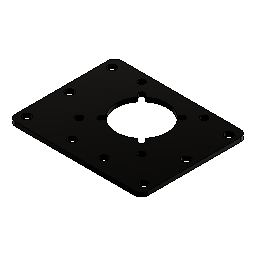
Router Concept v20 (Autodesk Fusion 360 archive; units mm, degrees)
design "Drive Module Bracket"
Autodesk Fusion 360 part; units mm, degrees
sketch "Dimension" plane through (0, 0, 0) normal (0, 1, 0) x (1, 0, 0)
  line L0 (50, -40) -> (-50, -40)
  line L1 (-50, -40) -> (-50, 40)
  line L2 (-50, 40) -> (50, 40)
  line L3 (50, 40) -> (50, -40)
  line L4 (50, -40) -> (-50, 40) construction
  line L5 (-50, -40) -> (50, 40) construction
  dimension "d4" = 100
  dimension "d5" = 80
  constraint horizontal L0
  constraint perpendicular L0 L1
  constraint parallel L0 L2
  constraint parallel L1 L3
  constraint coincident L4 origin
  constraint coincident L5 origin
  measures "d4" distance of L1.end L2.end
  measures "d5" distance of L0.end L1.end
extrude "Extrude1" add sketch "Dimension" along normal blind 3
sketch "Stepper Mount" plane through (0, 3, 0) normal (0, 1, 0) x (-1, 0, 0)
  line L0 (-50, -40) -> (50, -40)
  line L1 (50, -40) -> (50, 40)
  line L2 (50, 40) -> (-50, 40)
  line L3 (-50, 40) -> (-50, -40)
  line L4 (30, -40) -> (-30, -40)
  line L5 (-30, -40) -> (-30, 40) construction
  line L6 (-30, 40) -> (30, 40)
  line L7 (30, 40) -> (30, -40) construction
  circle A0 centre (23.55, -33.85) radius 2.55
  circle A1 centre (-23.55, -33.85) radius 2.55
  circle A2 centre (23.55, 13.25) radius 2.55
  circle A3 centre (-23.55, 13.25) radius 2.55
  line L8 (-23.55, 13.25) -> (23.55, -33.85)
  circle A4 centre (15.49, -25.79) radius 2
  line L9 (0, -10.3) -> (-30, -10.3) construction
  line L10 (0, -10.3) -> (0, -40) construction
  circle A5 centre (-15.49, -25.79) radius 2
  line L11 (15.49, -25.79) -> (-15.49, 5.19)
  line L12 (-15.49, 5.19) -> (-16.9042, 3.7758) construction
  line L13 (-16.9042, 3.7758) -> (14.0758, -27.2042)
  line L14 (14.0758, -27.2042) -> (15.49, -25.79)
  line L15 (15.49, -25.79) -> (-15.49, 5.19)
  line L16 (-15.49, 5.19) -> (-14.0758, 6.6042) construction
  line L17 (-14.0758, 6.6042) -> (16.9042, -24.3758)
  line L18 (16.9042, -24.3758) -> (15.49, -25.79)
  line L19 (14.0758, 6.6042) -> (-16.9042, -24.3758)
  line L20 (16.9042, 3.7758) -> (-14.0758, -27.2042)
  line L21 (23.55, 13.25) -> (13.5057, 3.2057) construction
  line L22 (1.4142, -8.8858) -> (-23.55, -33.85) construction
  arc A6 (16.9042, 3.7758) -> (14.0758, 6.6042) centre (15.49, 5.19) ccw
  arc A7 (-14.0758, 6.6042) -> (-16.9042, 3.7758) centre (-15.49, 5.19) ccw
  arc A8 (-13.5057, 3.2057) -> (-12.0173, 4.5457) centre (0, -10.3) ccw
  dimension "d8" = 60
  dimension "d9" = 38.2
  dimension "d10" = 30
  dimension "d11" = 29.7
  dimension "d12" = 5.1
  dimension "d13" = 6.45
  dimension "d14" = 6.15
  dimension "d15" = 5.1
  dimension "d16" = 6.15
  dimension "d17" = 53.55
  dimension "d18" = 5.1
  dimension "d19" = 6.45
  dimension "d20" = 53.25
  dimension "d21" = 5.1
  dimension "d22" = 53.25
  dimension "d23" = 53.55
  dimension "d24" = 14.51
  dimension "d25" = 14.21
  dimension "d26" = 4
  dimension "d27" = 2
  dimension "d28" = 2
  constraint horizontal L4
  constraint vertical L5
  constraint horizontal L6
  constraint vertical L7
  constraint midpoint L0 L4
  constraint collinear L2 L6
  constraint coincident A2.centre L21.start
  constraint coincident A1.centre L22.end
  constraint coincident A3.centre L8.start
  constraint coincident A0.centre L8.end
  constraint coincident L9.start L10.start
  constraint coincident L5 L9.end
  constraint perpendicular L5 L9
  constraint midpoint L4 L10.end
  constraint symmetric A4 L10 A5
  constraint symmetric A4 L9 A6
  constraint symmetric L9 A5 A7
  constraint perpendicular L11 L12
  constraint parallel L11 L13
  constraint parallel L12 L14
  constraint coincident L11.end L12.start
  constraint parallel L8 L11
  constraint coincident A4.centre L11.start
  constraint perpendicular L15 L16
  constraint parallel L15 L17
  constraint parallel L16 L18
  constraint perpendicular L12 L15
  constraint symmetric L10 L12.end L20.start
  constraint symmetric L10 L13.end L20.end
  constraint symmetric L10 L16.end L19.start
  constraint symmetric L10 L17.end L19.end
  constraint coincident L21.end A8
  constraint coincident L17 L22.start
  constraint collinear L21 L22
  constraint coincident L17 A8.end
  constraint coincident L8 A8.start
  measures "d8" distance of L4.start L4.end
  measures "d9" diameter of A8
  measures "d10" distance of L7 L9.start
  measures "d11" distance of L4 L9.start
  measures "d12" diameter of A0
  measures "d13" distance of L7 A0.centre
  measures "d14" distance of L4 A0.centre
  measures "d15" diameter of A1
  measures "d16" distance of L4 A1.centre
  measures "d17" distance of L7 A1.centre
  measures "d18" diameter of A2
  measures "d19" distance of L7 A2.centre
  measures "d20" distance of L4 A2.centre
  measures "d21" diameter of A3
  measures "d22" distance of L4 A3.centre
  measures "d23" distance of L7 A3.centre
  measures "d24" distance of L7 A4.centre
  measures "d25" distance of L4 A4.centre
  measures "d26" diameter of A4
  measures "d27" distance of A4.centre L13.end
  measures "d28" distance of A4.centre L17.end
extrude "Extrude2" cut sketch "Stepper Mount" against normal through all contours A0 | A1 | A2 | A3 | L8 L11 L15 L17 L19 A7 | L8 L11 L13 L15 A7 A8 | L8 L11 L13 L15 L19 A8 | L8 L11 L15 L17 L19 L20 | L8 L11 L13 L15 L19 L20 | L13 L19 A8 | L8 L11 L15 L17 L20 A8 | L8 L11 L13 L15 L20 A8 | L17 L19 L20 A8 | L17 L19 A8 | L13 L19 L20 A8 | A5 L19 L20 A8 | L8 A4 L11 L15 L17 A8 | L8 A4 L11 L13 L15 A8 | L17 L20 A8 | L13 L20 A8 | L19 L20 A6 A8 | A5 | L8 A4 L11 L15 L18 | L8 A4 L11 L14 L15 | L8 A4 L18 | L8 A4 L14
sketch "Idler Mount" plane through (0, 3, 0) normal (0, 1, 0) x (-1, 0, 0)
  circle A0 centre (23.55, 13.25) radius 2.55
  circle A1 centre (23.55, -33.85) radius 2.55
  line L0 (14.8457, -22.3173) -> (16.9042, -24.3758)
  arc A2 (14.0758, -27.2042) -> (16.9042, -24.3758) centre (15.49, -25.79) ccw
  line L1 (14.0758, -27.2042) -> (12.0173, -25.1457)
  arc A3 (-12.0173, -25.1457) -> (12.0173, -25.1457) centre (0, -10.3) ccw
  line L2 (-12.0173, -25.1457) -> (-14.0758, -27.2042)
  arc A4 (-16.9042, -24.3758) -> (-14.0758, -27.2042) centre (-15.49, -25.79) ccw
  line L3 (-16.9042, -24.3758) -> (-14.8457, -22.3173)
  arc A5 (-14.8457, 1.7173) -> (-14.8457, -22.3173) centre (0, -10.3) ccw
  line L4 (-14.8457, 1.7173) -> (-16.9042, 3.7758)
  arc A6 (-14.0758, 6.6042) -> (-16.9042, 3.7758) centre (-15.49, 5.19) ccw
  line L5 (-14.0758, 6.6042) -> (-12.0173, 4.5457)
  arc A7 (12.0173, 4.5457) -> (-12.0173, 4.5457) centre (0, -10.3) ccw
  line L6 (12.0173, 4.5457) -> (14.0758, 6.6042)
  arc A8 (16.9042, 3.7758) -> (14.0758, 6.6042) centre (15.49, 5.19) ccw
  line L7 (16.9042, 3.7758) -> (14.8457, 1.7173)
  arc A9 (14.8457, -22.3173) -> (14.8457, 1.7173) centre (0, -10.3) ccw
  circle A10 centre (-23.55, 13.25) radius 2.55
  circle A11 centre (-23.55, -33.85) radius 2.55
  line L8 (-50, -40) -> (50, -40)
  line L9 (50, -40) -> (50, 40)
  line L10 (50, 40) -> (-50, 40)
  line L11 (-50, 40) -> (-50, -40)
  arc A12 (-14.8457, 1.7173) -> (-14.8457, -22.3173) centre (0, -10.3) ccw
  arc A13 (-12.0173, -25.1457) -> (12.0173, -25.1457) centre (0, -10.3) ccw
  arc A14 (14.8457, -22.3173) -> (14.8457, 1.7173) centre (0, -10.3) ccw
  arc A15 (12.0173, 4.5457) -> (-12.0173, 4.5457) centre (0, -10.3) ccw
  circle A16 centre (0, -10.3) radius 6 construction
  line L12 (0, -10.3) -> (50, -10.3) construction
  line L13 (0, -10.3) -> (-50, -10.3) construction
  circle A17 centre (0, -10.3) radius 9
  line L14 (6, -10.3) -> (-6, -10.3)
  line L15 (-6, -10.3) -> (-6, 40) construction
  line L16 (-6, 40) -> (6, 40)
  line L17 (6, 40) -> (6, -10.3) construction
  line L18 (50, 30) -> (-50, 30) construction
  line L19 (-50, 30) -> (-50, 40)
  line L20 (-50, 40) -> (50, 40)
  line L21 (50, 40) -> (50, 30)
  circle A18 centre (12, 30) radius 6 construction
  circle A19 centre (12, 30) radius 9 construction
  circle A20 centre (12, 30) radius 3
  line L22 (0, 20) -> (0, 2.5)
  circle A21 centre (-12, 30) radius 9 construction
  circle A22 centre (-12, 30) radius 6 construction
  circle A23 centre (-12, 30) radius 3
  dimension "d30" = 12
  dimension "d31" = 18
  dimension "d33" = 10
  dimension "d38" = 12
  dimension "d39" = 18
  dimension "d41" = 6
  constraint concentric A15 A16
  constraint coincident A3.centre A5.centre
  constraint coincident L9 L12.end
  constraint perpendicular L9 L12
  constraint coincident L11 L13.end
  constraint perpendicular L11 L13
  constraint perpendicular L14 L15
  constraint parallel L14 L16
  constraint parallel L15 L17
  constraint coincident A16 L14.end
  constraint coincident L13 L14.end
  constraint parallel L13 L14
  constraint coincident A16 L14.start
  constraint horizontal L18
  constraint vertical L19
  constraint horizontal L20
  constraint vertical L21
  constraint collinear L11 L19
  constraint collinear L10 L20
  constraint collinear L9 L21
  constraint coincident L18 A18.centre
  constraint tangent L17 A18
  constraint concentric A18 A19
  constraint concentric A19 A20
  constraint symmetric A18 L22 A22
  constraint symmetric A19 L22 A21
  constraint symmetric A20 L22 A23
  measures "d30" diameter of A16
  measures "d31" diameter of A17
  measures "d33" distance of L18 L20
  measures "d38" diameter of A18
  measures "d39" diameter of A19
  measures "d41" diameter of A20
extrude "Extrude3" cut sketch "Idler Mount" against normal through all contours A20 | A23
sketch "Bracket Mount" plane through (0, 3, 0) normal (0, 1, 0) x (-1, 0, 0)
  circle A0 centre (12, 30) radius 3
  circle A1 centre (-12, 30) radius 3
  circle A2 centre (23.55, 13.25) radius 2.55
  circle A3 centre (23.55, -33.85) radius 2.55
  line L0 (14.8457, -22.3173) -> (16.9042, -24.3758)
  arc A4 (14.0758, -27.2042) -> (16.9042, -24.3758) centre (15.49, -25.79) ccw
  line L1 (14.0758, -27.2042) -> (12.0173, -25.1457)
  arc A5 (-12.0173, -25.1457) -> (12.0173, -25.1457) centre (0, -10.3) ccw
  line L2 (-12.0173, -25.1457) -> (-14.0758, -27.2042)
  arc A6 (-16.9042, -24.3758) -> (-14.0758, -27.2042) centre (-15.49, -25.79) ccw
  line L3 (-16.9042, -24.3758) -> (-14.8457, -22.3173)
  arc A7 (-14.8457, 1.7173) -> (-14.8457, -22.3173) centre (0, -10.3) ccw
  line L4 (-14.8457, 1.7173) -> (-16.9042, 3.7758)
  arc A8 (-14.0758, 6.6042) -> (-16.9042, 3.7758) centre (-15.49, 5.19) ccw
  line L5 (-14.0758, 6.6042) -> (-12.0173, 4.5457)
  arc A9 (12.0173, 4.5457) -> (-12.0173, 4.5457) centre (0, -10.3) ccw
  line L6 (12.0173, 4.5457) -> (14.0758, 6.6042)
  arc A10 (16.9042, 3.7758) -> (14.0758, 6.6042) centre (15.49, 5.19) ccw
  line L7 (16.9042, 3.7758) -> (14.8457, 1.7173)
  arc A11 (14.8457, -22.3173) -> (14.8457, 1.7173) centre (0, -10.3) ccw
  circle A12 centre (-23.55, 13.25) radius 2.55
  circle A13 centre (-23.55, -33.85) radius 2.55
  line L8 (-50, -40) -> (50, -40)
  line L9 (50, -40) -> (50, 40)
  line L10 (50, 40) -> (-50, 40)
  line L11 (-50, 40) -> (-50, -40)
  circle A14 centre (44, -32) radius 3.05
  line L12 (0, 20) -> (0, 2.5)
  circle A15 centre (-44, -32) radius 3.05
  line L13 (-2.5, 0) -> (-20, 0)
  circle A16 centre (44, 32) radius 3.05
  circle A17 centre (-44, 32) radius 3.05
  line L14 (-44, 32) -> (-44, -32) construction
  line L15 (44, -32) -> (44, 32) construction
  circle A18 centre (44, 0) radius 3.05
  circle A19 centre (-44, 0) radius 3.05
  dimension "d45" = 6.1
  dimension "d46" = 8
  dimension "d47" = 6
  dimension "d53" = 6.1
  constraint symmetric A14 L12 A15
  constraint symmetric A14 L13 A16
  constraint symmetric A15 L13 A17
  constraint coincident A17.centre L14.start
  constraint coincident A15.centre L14.end
  constraint coincident A14.centre L15.start
  constraint coincident A16.centre L15.end
  constraint midpoint L15 A18.centre
  constraint symmetric L12 A18 A19
  measures "d45" diameter of A14
  measures "d46" distance of L8 A14.centre
  measures "d47" distance of L9 A14.centre
  measures "d53" diameter of A18
extrude "Extrude4" cut sketch "Bracket Mount" against normal through all contours A14 | A15 | A16 | A17 | A18 | A19
fillet "Fillet1" radius 5 4 edges at (50, 1.5, -40) (-50, 1.5, -40) (-50, 1.5, 40) (50, 1.5, 40)
equation "PlateWidth = 100 mm"
equation "PlateHeight = 80 mm"
equation "PlateThickness = 3 mm"
equation "d4 = PlateWidth"
equation "d5 = PlateHeight"
equation "d6 = PlateThickness"
equation "IdlerToBaseDistance = 10 mm"
equation "d33 = IdlerToBaseDistance"
equation "IdlerInternalDiameter = 12 mm"
equation "IdlerOuterDiameter = 18 mm"
equation "DriverInnerDiameter = 12 mm"
equation "DriverOuterDiameter = 18 mm"
equation "d38 = IdlerInternalDiameter"
equation "d39 = IdlerOuterDiameter"
equation "IdlerBoreDiameter = 6 mm"
equation "d41 = IdlerBoreDiameter"
equation "BracketMountHoleDiameter = 6.1 mm"
equation "BracketMountHoleHDistance = 6 mm"
equation "d45 = BracketMountHoleDiameter"
equation "d46 = BracketMountHoleVDistance"
equation "d47 = BracketMountHoleHDistance"
equation "BracketFilletRadius = 5 mm"
equation "d51 = BracketFilletRadius"
equation "BracketMountHoleVDistance = 8 mm"
equation "d53 = BracketMountHoleDiameter"

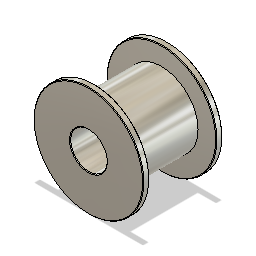
design "gt2 idler pulley 20T 10mm belt 6 mm bore"
Autodesk Fusion 360 part; units mm, degrees
sketch "Sketch1" plane through (0, 0, 0) normal (0, 1, 0) x (1, 0, 0)
  line L0 (0, 6.5) -> (9, 6.5)
  line L1 (9, 6.5) -> (9, -6.5)
  line L2 (9, -6.5) -> (0, -6.5)
  line L3 (0, -6.5) -> (0, 6.5)
  line L4 (6, 5.5) -> (9, 5.5)
  line L5 (9, 5.5) -> (9, -5.5)
  line L6 (9, -5.5) -> (6, -5.5)
  line L7 (6, -5.5) -> (6, 5.5)
  line L8 (0, 6.5) -> (3, 6.5)
  line L9 (3, 6.5) -> (3, -6.5)
  line L10 (3, -6.5) -> (0, -6.5)
  line L11 (0, -6.5) -> (0, 6.5)
  dimension "d1" = 9
  dimension "d2" = 13
  dimension "d3" = 3
  dimension "d4" = 11
  dimension "d5" = 3
  constraint horizontal L0
  constraint vertical L1
  constraint horizontal L2
  constraint vertical L3
  constraint midpoint origin L3
  constraint horizontal L4
  constraint vertical L5
  constraint horizontal L6
  constraint vertical L7
  constraint midpoint L1 L5
  constraint horizontal L8
  constraint vertical L9
  constraint horizontal L10
  constraint vertical L11
  constraint collinear L0 L8
  constraint collinear L2 L10
  constraint collinear L3 L11
  measures "d1" distance of L0.start L0.end
  measures "d2" distance of L0.start L2.end
  measures "d3" distance of L4.start L4.end
  measures "d4" distance of L4.start L6.end
  measures "d5" distance of L0.start L8.end
revolve "Revolve1" add sketch "Sketch1" angle 360 about axis through (0, 0, 6.5) along (0, 0, -1) contours L0 L1 L2 L4 L6 L7 L9
chamfer "Chamfer1" distance 0.1 angle 45 1 edges at (-8.3909, -3.2545, 6.5)
chamfer "Chamfer2" distance 0.1 angle 45 5 edges at (-2.797, -1.0848, 6.5) (-8.3909, -3.2545, 5.5) (-8.3909, -3.2545, -5.5) (-8.3909, -3.2545, -6.5) (-2.797, -1.0848, -6.5)
